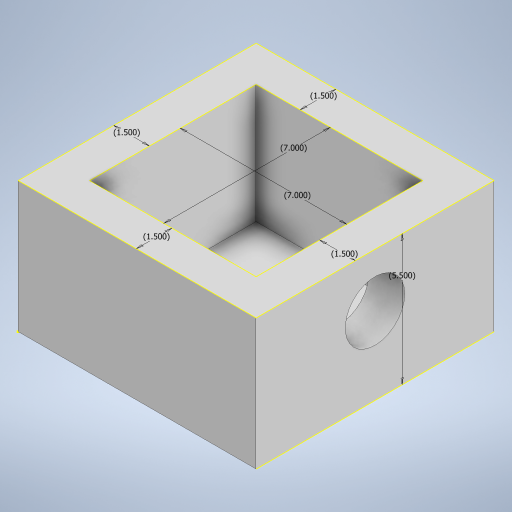
# Autodesk Inventor part: Vacuum_Box
Saved by Autodesk Inventor 2023 (Build 270158000, 158)
## iProperties
Created: 2022-10-03
Part Number: Vacuum_Box
Material: Generic
Document SubType Name: Modeling
Designer: myers
Density: 1 g/cm^3
Appearance: Default
Author: myers
Autodesk Inventor part; units mm, degrees
ref_plane "YZ Plane" through (0, 0, 0) normal (1, 0, 0) x (0, 1, 0)
ref_plane "XZ Plane" through (0, 0, 0) normal (0, 1, 0) x (-1, 0, 0)
ref_plane "XY Plane" through (0, 0, 0) normal (0, 0, 1) x (1, 0, 0)
sketch "Sketch1" plane through (0, 0, 0) normal (0, 1, 0) x (-1, 0, 0)
  line L0 (0, 0) -> (254, 0)
  line L1 (254, 0) -> (254, -254)
  line L2 (254, -254) -> (0, -254)
  line L3 (0, -254) -> (0, 0)
  dimension "d0" = 254
  dimension "d1" = 254
  constraints: 8 end point, 2 parallel, 1 horizontal, 1 perpendicular
  measures "d0" distance of L0.end L1.end
  measures "d1" distance of L1.end L2.end
extrude "Extrusion1" add sketch "Sketch1" along normal blind 12.7
sketch "Sketch2" plane through (0, 12.7, 0) normal (0, 1, 0) x (1, 0, 0)
  line L0 (-25.4, 25.4) -> (-228.6, 25.4)
  line L1 (-228.6, 25.4) -> (-228.6, 228.6)
  line L2 (-228.6, 228.6) -> (-25.4, 228.6)
  line L3 (-25.4, 228.6) -> (-25.4, 25.4)
  line L4 (-254, 254) -> (-254, 0) projected
  line L5 (0, 254) -> (-254, 254) projected
  line L6 (-254, 0) -> (0, 0) projected
  line L7 (0, 0) -> (0, 254) projected
  point P0 (0, 127)
  dimension "d8" = 25.4
  dimension "d9" = 25.4
  dimension "d10" = 25.4
  dimension "d11" = 25.4
  constraints: 8 end point, 2 parallel, 1 horizontal, 1 midpoint, 1 perpendicular
  measures "d8" distance between parallel lines of L4 L1
  measures "d9" distance between parallel lines of L5 L2
  measures "d10" distance between parallel lines of L6 L0
  measures "d11" distance from line of point (0, 127) L3
extrude "Extrusion2" add sketch "Sketch2" along normal blind 127 contours L0 L1 L2 L3
shell "Shell1" thickness 12.7 removed faces 1 at (-93.1333, 139.7, -93.1333)
sketch "Sketch4" plane through (0, 12.7, 0) normal (0, 1, 0) x (1, 0, 0)
  line L0 (0, 0) -> (0, 254) projected
  line L1 (0, 254) -> (-254, 254) projected
  line L2 (0, 0) -> (-254, 0)
  line L3 (-254, 0) -> (-254, 254)
  line L4 (-254, 254) -> (0, 254)
  line L5 (0, 254) -> (0, 0)
  line L6 (-25.4, 25.4) -> (-25.4, 228.6) projected
  line L7 (-228.6, 228.6) -> (-228.6, 25.4) projected
  line L8 (-25.4, 25.4) -> (-228.6, 25.4)
  line L9 (-228.6, 25.4) -> (-228.6, 228.6)
  line L10 (-228.6, 228.6) -> (-25.4, 228.6)
  line L11 (-25.4, 228.6) -> (-25.4, 25.4)
  constraints: 16 end point, 4 parallel, 2 horizontal, 2 perpendicular
extrude "Extrusion3" add sketch "Sketch4" along normal blind 127
sketch "Sketch5" plane through (0, 139.7, 0) normal (0, 1, 0) x (1, 0, 0)
  line L0 (-38.1, 38.1) -> (-215.9, 38.1) projected
  line L1 (-254, 0) -> (0, 0) projected
  line L2 (-38.1, 215.9) -> (-38.1, 38.1) projected
  line L3 (-215.9, 38.1) -> (-215.9, 215.9) projected
  line L4 (-215.9, 215.9) -> (-38.1, 215.9) projected
  line L5 (0, 254) -> (-254, 254) projected
  line L6 (0, 0) -> (0, 254) projected
  line L7 (-254, 254) -> (-254, 0) projected
  dimension "d17" = 38.1
  dimension "d18" = 177.8
  dimension "d19" = 177.8
  dimension "d20" = 38.1
  dimension "d21" = 38.1
  dimension "d22" = 38.1
  measures "d17" distance between parallel lines of L0 L1
  measures "d18" distance between parallel lines of L2 L3
  measures "d19" distance between parallel lines of L4 L0
  measures "d20" distance between parallel lines of L5 L4
  measures "d21" distance between parallel lines of L6 L2
  measures "d22" distance between parallel lines of L7 L3
sketch "Sketch6" plane through (0, 0, 0) normal (1, 0, 0) x (0, 0, -1)
  line L0 (0, 0) -> (254, 0) projected
  line L1 (0, 139.7) -> (254, 139.7) projected
  dimension "d23" = 139.7
  measures "d23" distance between parallel lines of L0 L1
sketch "Sketch7" plane through (-254, 0, -254) normal (-1, 0, 0) x (0, 0, 1)
  point P0 (254, 0)
sketch "Sketch8" plane through (0, 0, 0) normal (1, 0, 0) x (0, 0, -1)
  line L0 (0, 139.7) -> (254, 139.7) projected
  line L1 (254, 0) -> (254, 139.7) projected
  circle A0 centre (127, 82.55) radius 31.75
  point P0 (0, 0)
  dimension "d24" = 57.15
  dimension "d25" = 127
  dimension "d26" = 63.5
  constraints: 1 centre point, 1 coincident
  measures "d24" distance from line of L0 point (127, 82.55)
  measures "d25" distance from line of L1 point (127, 82.55)
  measures "d26" diameter of A0
extrude "Extrusion4" cut sketch "Sketch8" against normal blind 50.8
body "Solid1"
